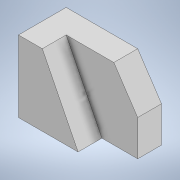
# Autodesk Inventor part: 7.1 Part 4
Saved by Autodesk Inventor 2020 (Build 240168000, 168)
## iProperties
Created: 2020-03-12
Part Number: 7.1 Part 4
Material: Generic
Document SubType Name: Modeling
Designer: cks4a449
Density: 1 g/cm^3
Appearance: Default
Author: cks4a449
Autodesk Inventor part; units mm, degrees
ref_plane "YZ Plane" through (0, 0, 0) normal (1, 0, 0) x (0, 1, 0)
ref_plane "XZ Plane" through (0, 0, 0) normal (0, 1, 0) x (-1, 0, 0)
ref_plane "XY Plane" through (0, 0, 0) normal (0, 0, 1) x (1, 0, 0)
sketch "Sketch1" plane through (0, 0, 0) normal (0, 1, 0) x (-1, 0, 0)
  line L0 (0, -12.7) -> (0, -25.4)
  line L1 (0, -25.4) -> (50.8, -25.4)
  line L2 (50.8, -25.4) -> (50.8, 0)
  line L3 (50.8, 0) -> (19.05, 0)
  line L4 (19.05, 0) -> (19.05, -12.7)
  line L5 (19.05, -12.7) -> (0, -12.7)
  point P0 (0, 0)
  dimension "d0" = 12.7
  dimension "d1" = 50.8
  dimension "d2" = 25.4
  dimension "d3" = 31.75
  dimension "d4" = 12.7
  constraints: 12 end point, 4 perpendicular, 1 vertical
  measures "d0" distance of L0.start L0.end
  measures "d1" distance of L0.end L1.end
  measures "d2" distance of L1.end L2.end
  measures "d3" distance of L2.end L3.end
  measures "d4" distance of L3.end L4.end
extrude "Extrusion1" add sketch "Sketch1" along normal blind 38.1
chamfer "Chamfer1" distance 19.05 distance2 38.1 1 edges at (-19.05, 38.1, -6.35) measured on face at (-40.2167, 38.1, -12.7)
chamfer "Chamfer2" distance 12.7 distance2 19.05 1 edges at (0, 38.1, -19.05) measured on face at (-23.2833, 38.1, -21.1667)
body "Solid1"
